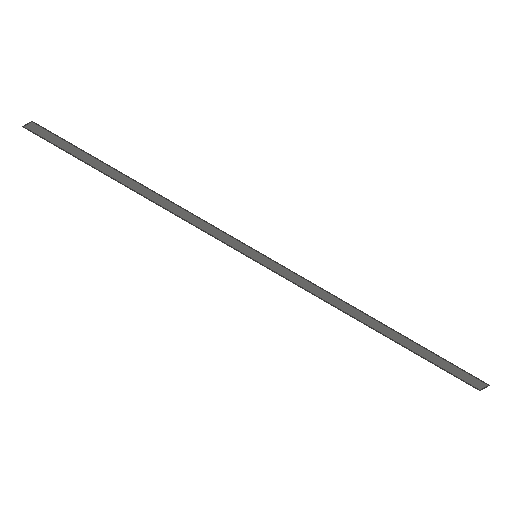
# Autodesk Inventor part: pasek ledów os x 410mm
Saved by Autodesk Inventor 2026.1 (Build 301233000, 233)
## iProperties
Created: 2016-06-18
Part Number: pasek ledów os x 410mm
Material: Ogólny
Document SubType Name: Modeling
Designer: Andrzej
Density: 1 g/cm^3
Appearance: Szara
Mass: 0.9576 g
Surface Area: 66.282 cm^2
Volume: 0.9576 cm^3
Author: Andrzej
Autodesk Inventor part; units mm, degrees
ref_plane "YZ Plane" through (0, 0, 0) normal (1, 0, 0) x (0, 1, 0)
ref_plane "XZ Plane" through (0, 0, 0) normal (0, 1, 0) x (-1, 0, 0)
ref_plane "XY Plane" through (0, 0, 0) normal (0, 0, 1) x (1, 0, 0)
sketch "Szkic1" plane through (0, 0, 0) normal (0, 0, 1) x (1, 0, 0)
  line L0 (-7.6889, 6.8896) -> (391.3111, 6.8896)
  line L1 (391.3111, 6.8896) -> (391.3111, -1.1104)
  line L2 (391.3111, -1.1104) -> (-7.6889, -1.1104)
  line L3 (-7.6889, -1.1104) -> (-7.6889, 6.8896)
  point P0 (0, 0)
  dimension "d0" = 399
  dimension "d1" = 8
  constraints: 8 end point, 2 parallel, 1 horizontal, 1 perpendicular
  measures "d0" distance of L1.end L2.end
  measures "d1" distance of L0.end L1.end
extrude "Wyciągnięcie proste1" add sketch "Szkic1" along normal blind 0.3
